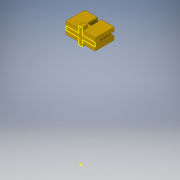
# Autodesk Inventor part: Aligner Helper v1
Saved by Autodesk Inventor 2019 (Build 230136000, 136)
## iProperties
Created: 2021-08-08
Part Number: Aligner Helper v1
Material: Generic
Document SubType Name: Modeling
Designer: Lix
Density: 1 g/cm^3
Appearance: Gold
Author: Lix
## iProperties of the stored document Aligner Helper v1_3DPrint.ipt
Created: 2021-08-08
Part Number: Aligner Helper v1_3DPrint
Material: Generic
Document SubType Name: Modeling
Designer: Lix
Density: 1 g/cm^3
Appearance: Default
Author: Lix
Autodesk Inventor part; units mm, degrees
ref_plane "YZ Plane" through (0, 0, 0) normal (1, 0, 0) x (0, 1, 0)
ref_plane "XZ Plane" through (0, 0, 0) normal (0, 1, 0) x (-1, 0, 0)
ref_plane "XY Plane" through (0, 0, 0) normal (0, 0, 1) x (1, 0, 0)
sketch "Sketch1" plane through (0, 0, 0) normal (0, 0, 1) x (1, 0, 0)
  line L0 (-1.5, 81) -> (1.5, 81) projected
  line L1 (1.5, 81) -> (1.5, 86) projected
  line L2 (-1.5, 86) -> (1.5, 86) projected
  line L3 (-1.5, 86) -> (-1.5, 81) projected
  arc A0 (-53.4049, -82.5) -> (-44.7446, -87.5) centre (-44.7446, -77.5) ccw projected
  line L4 (-44.7446, -87.5) -> (44.7446, -87.5) projected
  arc A1 (44.7446, -87.5) -> (53.4049, -82.5) centre (44.7446, -77.5) ccw projected
  line L5 (53.4049, -82.5) -> (98.1495, -5) projected
  arc A2 (98.1495, -5) -> (98.1495, 5) centre (89.4893, 0) ccw projected
  line L6 (98.1495, 5) -> (53.4049, 82.5) projected
  arc A3 (53.4049, 82.5) -> (44.7446, 87.5) centre (44.7446, 77.5) ccw projected
  line L7 (44.7446, 87.5) -> (-44.7446, 87.5) projected
  arc A4 (-44.7446, 87.5) -> (-53.4049, 82.5) centre (-44.7446, 77.5) ccw projected
  line L8 (-53.4049, 82.5) -> (-98.1495, 5) projected
  arc A5 (-98.1495, 5) -> (-98.1495, -5) centre (-89.4893, 0) ccw projected
  line L9 (-98.1495, -5) -> (-53.4049, -82.5) projected
  line L10 (-50.8068, -84) -> (-98.1495, -2) projected
  arc A6 (-98.1495, 2) -> (-98.1495, -2) centre (-94.6854, 0) ccw projected
  line L11 (-98.1495, 2) -> (-50.8068, 84) projected
  arc A7 (-47.3427, 86) -> (-50.8068, 84) centre (-47.3427, 82) ccw projected
  line L12 (-47.3427, 86) -> (47.3427, 86) projected
  arc A8 (50.8068, 84) -> (47.3427, 86) centre (47.3427, 82) ccw projected
  line L13 (50.8068, 84) -> (98.1495, 2) projected
  arc A9 (98.1495, -2) -> (98.1495, 2) centre (94.6854, 0) ccw projected
  line L14 (98.1495, -2) -> (50.8068, -84) projected
  arc A10 (47.3427, -86) -> (50.8068, -84) centre (47.3427, -82) ccw projected
  line L15 (47.3427, -86) -> (-47.3427, -86) projected
  arc A11 (-50.8068, -84) -> (-47.3427, -86) centre (-47.3427, -82) ccw projected
  line L16 (47.3427, 89) -> (-47.3427, 89) projected
  line L17 (1.5, 94) -> (-1.5, 94) projected
  line L18 (-1.5, 94) -> (-1.5, 89) projected
  line L19 (1.5, 89) -> (-1.5, 89) projected
  line L20 (1.5, 89) -> (1.5, 94) projected
  line L21 (1.5, 97) -> (1.5, 94) projected
  line L22 (-1.5, 97) -> (1.5, 97) projected
  line L23 (-1.5, 94) -> (-1.5, 97) projected
  line L24 (1.5, 94) -> (-1.5, 94) projected
  line L25 (-1.5, 78) -> (-1.5, 81) projected
  line L26 (1.5, 78) -> (-1.5, 78) projected
  line L27 (1.5, 81) -> (1.5, 78) projected
  line L28 (-1.5, 81) -> (1.5, 81) projected
  line L29 (-11.5, 89) -> (11.5, 89)
  line L30 (11.5, 89) -> (11.5, 86)
  line L31 (11.5, 86) -> (-11.5, 86)
  line L32 (-11.5, 86) -> (-11.5, 89)
  line L33 (1.5, 92) -> (1.5, 83)
  line L34 (-1.5, 83) -> (-1.5, 92)
  line L35 (1.5, 92) -> (-1.5, 92)
  line L36 (1.5, 83) -> (-1.5, 83)
  point P0 (0, 0)
  dimension "d0" = 10
  dimension "d1" = 10
  dimension "d14" = 3
  dimension "d15" = 3
  constraints: 16 end point, 3 parallel, 3 perpendicular, 2 point on line, 1 horizontal
  measures "d0" distance between parallel lines of L32 L18
  measures "d1" distance between parallel lines of L20 L30
  measures "d14" distance between parallel lines of L16 L35
  measures "d15" distance between parallel lines of L36 L2
extrude "Extrusion1" add sketch "Sketch1" along normal blind 4 contours L3 L36 L1 L0 | L3 L2 L1 L36 | L34 L7 L33 L2 | L12 L32 L7 L34 | L33 L7 L30 L12 | L34 L16 L33 L7 | L7 L32 L16 L34 | L33 L16 L30 L7 | L18 L35 L20 L16 | L18 L17 L20 L35
sketch "Sketch2" plane through (0, 0, 4) normal (0, 0, 1) x (1, 0, 0)
  line L0 (1.5, 81) -> (1.5, 86) projected
  line L1 (1.5, 86) -> (11.5, 86) projected
  line L2 (11.5, 86) -> (11.5, 89) projected
  line L3 (11.5, 89) -> (1.5, 89) projected
  line L4 (1.5, 89) -> (1.5, 94) projected
  line L5 (-1.5, 94) -> (-1.5, 89) projected
  line L6 (-1.5, 89) -> (-11.5, 89) projected
  line L7 (-11.5, 89) -> (-11.5, 86) projected
  line L8 (-11.5, 86) -> (-1.5, 86) projected
  line L9 (-1.5, 86) -> (-1.5, 81) projected
  line L10 (-1.5, 81) -> (1.5, 81) projected
  line L11 (1.5, 94) -> (-1.5, 94) projected
  point P0 (0, 0)
sketch "Sketch3" plane through (0, 0, 4) normal (0, 0, 1) x (1, 0, 0)
  line L0 (11.5, 92) -> (-11.5, 92)
  line L1 (-11.5, 92) -> (-11.5, 83)
  line L2 (-11.5, 83) -> (11.5, 83)
  line L3 (11.5, 83) -> (11.5, 92)
  line L4 (11.5, 86) -> (11.5, 89) projected
  line L5 (-11.5, 89) -> (-11.5, 86) projected
  line L6 (1.5, 86) -> (11.5, 86) projected
  line L7 (11.5, 89) -> (1.5, 89) projected
  line L8 (-1.5, 86) -> (-11.5, 86)
  line L9 (-11.5, 86) -> (-11.5, 83)
  line L10 (-11.5, 83) -> (-1.5, 83)
  line L11 (-1.5, 83) -> (-1.5, 86)
  line L12 (-11.5, 89) -> (-11.5, 86) projected
  line L13 (-1.5, 92) -> (-11.5, 92)
  line L14 (-11.5, 92) -> (-11.5, 89)
  line L15 (-11.5, 89) -> (-1.5, 89)
  line L16 (-1.5, 89) -> (-1.5, 92)
  line L17 (-1.5, 94) -> (-1.5, 89) projected
  line L18 (1.5, 81) -> (1.5, 86) projected
  line L19 (11.5, 83) -> (1.5, 83)
  line L20 (1.5, 83) -> (1.5, 86)
  line L21 (1.5, 86) -> (11.5, 86)
  line L22 (11.5, 86) -> (11.5, 83)
  line L23 (11.5, 89) -> (1.5, 89)
  line L24 (1.5, 89) -> (1.5, 92)
  line L25 (1.5, 92) -> (11.5, 92)
  line L26 (11.5, 92) -> (11.5, 89)
  point P0 (0, 0)
  point P1 (-1.5, 97)
  point P2 (1.5, 78)
  dimension "d4" = 3
  dimension "d5" = 3
  constraints: 40 end point, 10 parallel, 5 horizontal, 5 perpendicular, 4 point on line, 3 collinear
  measures "d4" distance between parallel lines of L2 L6
  measures "d5" distance between parallel lines of L0 L7
extrude "Extrusion2" add sketch "Sketch3" against normal blind 15 contours L3 L7 L24 L0 | L16 L15 L1 L0 | L3 L2 L18 L6 | L8 L11 L2 L1
sketch "Sketch4" plane through (0, 0, 0) normal (0, 0, -1) x (-1, 0, 0)
  line L0 (-1.5, 89) -> (-1.5, 92) projected
  line L1 (-11.5, 89) -> (-1.5, 89) projected
  line L2 (-11.5, 86) -> (-11.5, 89) projected
  line L3 (-1.5, 86) -> (-11.5, 86) projected
  line L4 (-1.5, 83) -> (-1.5, 86) projected
  line L5 (-1.5, 81) -> (-1.5, 83) projected
  line L6 (1.5, 83) -> (1.5, 81) projected
  line L7 (1.5, 86) -> (1.5, 83) projected
  line L8 (11.5, 86) -> (1.5, 86) projected
  line L9 (11.5, 89) -> (11.5, 86) projected
  line L10 (1.5, 89) -> (11.5, 89) projected
  line L11 (1.5, 92) -> (1.5, 89) projected
  line L12 (1.5, 94) -> (1.5, 92) projected
  line L13 (-1.5, 92) -> (-1.5, 94) projected
  line L14 (-1.5, 83) -> (-1.5, 86) projected
  line L15 (-1.5, 86) -> (-11.5, 86) projected
  line L16 (-11.5, 86) -> (-11.5, 83) projected
  line L17 (-11.5, 83) -> (-1.5, 83) projected
  line L18 (-1.5, 89) -> (-1.5, 92) projected
  line L19 (-1.5, 92) -> (-11.5, 92) projected
  line L20 (-11.5, 92) -> (-11.5, 89) projected
  line L21 (-11.5, 89) -> (-1.5, 89) projected
  line L22 (1.5, 89) -> (11.5, 89) projected
  line L23 (11.5, 89) -> (11.5, 92) projected
  line L24 (11.5, 92) -> (1.5, 92) projected
  line L25 (1.5, 92) -> (1.5, 89) projected
  line L26 (11.5, 83) -> (11.5, 86) projected
  line L27 (11.5, 86) -> (1.5, 86) projected
  line L28 (1.5, 86) -> (1.5, 83) projected
  line L29 (1.5, 83) -> (11.5, 83) projected
  line L30 (-1.5, 89) -> (-1.5, 92) projected
  line L31 (1.5, 89) -> (-1.5, 89)
  line L32 (-1.5, 89) -> (-1.5, 92)
  line L33 (-1.5, 92) -> (1.5, 92)
  line L34 (1.5, 92) -> (1.5, 89)
  line L35 (-1.5, 83) -> (-1.5, 86) projected
  line L36 (1.5, 86) -> (-1.5, 86)
  line L37 (-1.5, 86) -> (-1.5, 83)
  line L38 (-1.5, 83) -> (1.5, 83)
  line L39 (1.5, 83) -> (1.5, 86)
  line L40 (1.5, 81) -> (-1.5, 81) projected
  line L41 (-1.5, 94) -> (1.5, 94) projected
  point P0 (0, 0)
  dimension "d8" = 3
  dimension "d9" = 3
  dimension "d10" = 3
  dimension "d11" = 3
  constraints: 16 end point, 4 parallel, 2 horizontal, 2 perpendicular
  measures "d8" distance of L18.end L33.end
  measures "d9" distance of L31.end L18.end
  measures "d10" distance of L38.end L14.start
  measures "d11" distance of L14.start L36.end
extrude "Extrusion3" add sketch "Sketch4" along normal blind 3 contours L0 L33 L11 L31 | L36 L7 L38 L4
equation "\"d1\" = d0"
equation "\"d15\" = d14"
equation "\"d5\" = d4"
body "Solid1"
